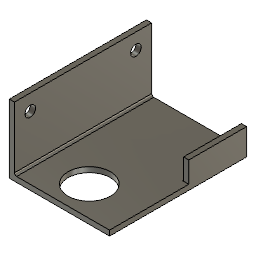
PlateCam_Shelf (Autodesk Fusion 360 design; units mm, degrees)
Autodesk Fusion 360 part; units mm, degrees
sketch "Sketch1" plane through (0, 0, 0) normal (0, 0, 1) x (1, 0, 0)
  line L0 (-45, 60) -> (45, 60)
  line L1 (45, 60) -> (45, -60)
  line L2 (45, -60) -> (-45, -60)
  line L3 (-45, -60) -> (-45, 60)
  line L4 (-45, 60) -> (45, -60) construction
  line L5 (45, 60) -> (-45, -60) construction
  dimension "d1" = 90
  dimension "d2" = 120
  constraint horizontal L0
  constraint perpendicular L0 L1
  constraint parallel L0 L2
  constraint parallel L1 L3
  constraint coincident L4 origin
  constraint coincident L5 origin
  measures "d1" distance of L1.end L2.end
  measures "d2" distance of L0.end L1.end
sketch "Sketch3" plane through (0, 0, 0) normal (0, 0, 1) x (1, 0, 0)
  line L0 (-47.5, 65) -> (47.5, 65)
  line L1 (47.5, 65) -> (47.5, -65)
  line L2 (47.5, -65) -> (-47.5, -65)
  line L3 (-47.5, -65) -> (-47.5, 65)
  line L4 (-47.5, 65) -> (47.5, -65) construction
  line L5 (47.5, 65) -> (-47.5, -65) construction
  dimension "d8" = 95
  dimension "d9" = 130
  constraint horizontal L0
  constraint perpendicular L0 L1
  constraint parallel L0 L2
  constraint parallel L1 L3
  constraint coincident L4 origin
  constraint coincident L5 origin
  measures "d8" distance of L1.end L2.end
  measures "d9" distance of L0.end L1.end
extrude "Extrude3" add sketch "Sketch3" along normal blind 5
sketch "Sketch4" plane through (0, 0, 5) normal (0, 0, 1) x (-1, 0, 0)
  line L0 (47.5, 65) -> (-47.5, 65)
  line L1 (-47.5, 65) -> (-47.5, -65)
  line L2 (-47.5, -65) -> (47.5, -65)
  line L3 (47.5, -65) -> (47.5, 65)
  circle A0 centre (0, 36.6491) radius 20
  dimension "d12" = 40
  measures "d12" diameter of A0
extrude "Extrude4" cut sketch "Sketch4" against normal blind 10 contours A0
sketch "Sketch5" plane through (0, 0, 5) normal (0, 0, 1) x (-1, 0, 0)
  circle A0 centre (0, 36.6491) radius 20
  line L0 (47.5, 65) -> (-47.5, 65)
  line L1 (-47.5, 65) -> (-47.5, -65)
  line L2 (-47.5, -65) -> (47.5, -65)
  line L3 (47.5, -65) -> (47.5, 65)
  line L4 (47.5, -65) -> (42.5, -65)
  line L5 (42.5, -65) -> (42.5, 65)
  line L6 (42.5, 65) -> (47.5, 65)
  line L7 (47.5, 65) -> (47.5, -65)
  dimension "d15" = 5
  constraint horizontal L4
  constraint vertical L5
  constraint horizontal L6
  constraint vertical L7
  constraint coincident L0 L5.end
  constraint coincident L2.end L3.start
  measures "d15" distance of L2.end L4.end
extrude "Extrude5" add sketch "Sketch5" along normal blind 60 contours L0 L2 L3 L4 L5 L6 L7
fillet "Fillet1" radius 2 1 edges at (-42.5, 0, 5)
sketch "Sketch6" plane through (-42.5, 0, 0) normal (1, 0, 0) x (0, 1, 0)
  line L0 (-65, 7) -> (65, 7)
  line L1 (65, 7) -> (65, 65)
  line L2 (65, 65) -> (-65, 65)
  line L3 (-65, 65) -> (-65, 7)
  circle A0 centre (-50, 50) radius 5
  circle A1 centre (50, 50) radius 5
  dimension "d20" = 10
  dimension "d21" = 10
  measures "d20" diameter of A0
  measures "d21" diameter of A1
extrude "Extrude6" cut sketch "Sketch6" against normal blind 10 contours A0
sketch "Sketch7" plane through (-42.5, 0, 0) normal (1, 0, 0) x (0, 1, 0)
  circle A0 centre (-50, 50) radius 5
  line L0 (-65, 7) -> (65, 7)
  line L1 (65, 7) -> (65, 65)
  line L2 (65, 65) -> (-65, 65)
  line L3 (-65, 65) -> (-65, 7)
  circle A1 centre (50, 50) radius 5
  dimension "d24" = 10
  measures "d24" diameter of A1
extrude "Extrude7" cut sketch "Sketch7" against normal blind 20 contours A1
sketch "Sketch8" plane through (0, 0, 5) normal (0, 0, 1) x (-1, 0, 0)
  line L0 (40.5, -65) -> (40.5, 65)
  line L1 (40.5, 65) -> (-47.5, 65)
  line L2 (-47.5, 65) -> (-47.5, -65)
  line L3 (-47.5, -65) -> (40.5, -65)
  circle A0 centre (0, 36.6491) radius 20
  line L4 (-47.5, -10.1158) -> (-42.5, -10.1158)
  line L5 (-42.5, -10.1158) -> (-42.5, -65)
  line L6 (-42.5, -65) -> (-47.5, -65)
  line L7 (-47.5, -65) -> (-47.5, -10.1158)
  dimension "d27" = 5
  constraint horizontal L4
  constraint vertical L5
  constraint horizontal L6
  constraint vertical L7
  constraint coincident L2 L4.start
  measures "d27" distance of L4.start L4.end
extrude "Extrude8" add sketch "Sketch8" along normal blind 20 contours L2 L3 L4 L5 L6 L7
fillet "Fillet2" radius 1 1 edges at (42.5, 37.5579, 5)
extrude "Extrude1" [suppressed]
sketch "Sketch2" plane through (0, 0, 5) normal (0, 0, 1) x (-1, 0, 0)
  line L0 (45, 60) -> (-45, 60)
  line L1 (-45, 60) -> (-45, -60)
  line L2 (-45, -60) -> (45, -60)
  line L3 (45, -60) -> (45, 60)
  circle A0 centre (0, 0) radius 20
  dimension "d5" = 40
  constraint coincident A0.centre origin
  measures "d5" diameter of A0
extrude "Extrude2" [suppressed]
